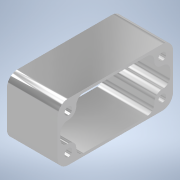
# Autodesk Inventor part: NASA-20-MM-MP-01
Saved by Autodesk Inventor 2020 (Build 240168000, 168)
## iProperties
Created: 2019-09-22
Part Number: NASA-20-MM-MP-01
Material: Aluminum 6061
Document SubType Name: Modeling
Designer: Rick Szalay
Density: 2.7 g/cm^3
Appearance: Aluminum - Flat
Description: MOUNTING BLOCK
Author: Rick Szalay
Autodesk Inventor part; units mm, degrees
ref_plane "YZ Plane" through (0, 0, 0) normal (1, 0, 0) x (0, 1, 0)
ref_plane "XZ Plane" through (0, 0, 0) normal (0, 1, 0) x (-1, 0, 0)
ref_plane "XY Plane" through (0, 0, 0) normal (0, 0, 1) x (1, 0, 0)
sketch "Sketch1" plane through (0, 0, 0) normal (1, 0, 0) x (0, 1, 0)
  line L0 (-25.4, -50.8) -> (25.4, -50.8)
  line L1 (25.4, -50.8) -> (25.4, 50.8)
  line L2 (25.4, 50.8) -> (-25.4, 50.8)
  line L3 (-25.4, 50.8) -> (-25.4, -50.8)
  line L4 (-25.4, -50.8) -> (25.4, 50.8) construction
  line L5 (25.4, -50.8) -> (-25.4, 50.8) construction
  point P0 (0, 0)
  dimension "d0" = 50.8
  dimension "d1" = 101.6
  constraints: 12 end point, 2 midpoint, 2 parallel, 1 horizontal, 1 perpendicular
  measures "d0" distance of L0.start L0.end
  measures "d1" distance between parallel lines of L2 L0
extrude "Extrusion1" add sketch "Sketch1" along normal blind 44.45
fillet "Fillet2" radius 9.525 4 edges at (22.225, 25.4, 50.8) (22.225, -25.4, 50.8) (22.225, -25.4, -50.8) (22.225, 25.4, -50.8)
sketch "Sketch5" plane through (44.45, 0, 0) normal (1, 0, 0) x (0, 0, -1)
  arc A0 (50.8, 15.875) -> (41.275, 25.4) centre (41.275, 15.875) ccw projected
  line L0 (41.275, 25.4) -> (-41.275, 25.4) projected
  arc A1 (-41.275, 25.4) -> (-50.8, 15.875) centre (-41.275, 15.875) ccw projected
  line L1 (-50.8, 15.875) -> (-50.8, -15.875) projected
  arc A2 (-50.8, -15.875) -> (-41.275, -25.4) centre (-41.275, -15.875) ccw projected
  line L2 (-41.275, -25.4) -> (41.275, -25.4) projected
  arc A3 (41.275, -25.4) -> (50.8, -15.875) centre (41.275, -15.875) ccw projected
  line L3 (50.8, -15.875) -> (50.8, 15.875) projected
  point P0 (0, 0)
hole "Hole2" at (44.45, -15.875, -41.275) at (44.45, -15.875, 41.275) at (44.45, 15.875, 41.275) at (44.45, 15.875, -41.275) direction (-1, 0, 0) diameter 6.7564 end through all clearance for "Flat Head Machine Screw (82)" size "1/4" standard "Ansi Unified Screw Threads"
sketch "Sketch6" plane through (44.45, 0, 0) normal (1, 0, 0) x (0, 0, -1)
  circle A0 centre (41.275, -15.875) radius 3.3782 projected
  circle A1 centre (41.275, -15.875) radius 6.985
  circle A2 centre (41.275, 15.875) radius 3.3782 projected
  circle A3 centre (41.275, 15.875) radius 6.985
  circle A4 centre (-41.275, 15.875) radius 3.3782 projected
  circle A5 centre (-41.275, 15.875) radius 6.985
  circle A6 centre (-41.275, -15.875) radius 3.3782 projected
  circle A7 centre (-41.275, -15.875) radius 6.985
  line L0 (-48.26, 22.86) -> (48.26, 22.86)
  line L1 (48.26, 22.86) -> (48.26, -22.86)
  line L2 (48.26, -22.86) -> (-48.26, -22.86)
  line L3 (-48.26, -22.86) -> (-48.26, 22.86)
  line L4 (-48.26, 22.86) -> (48.26, -22.86) construction
  line L5 (48.26, 22.86) -> (-48.26, -22.86) construction
  arc A8 (41.275, -25.4) -> (50.8, -15.875) centre (41.275, -15.875) ccw projected
  arc A9 (50.8, 15.875) -> (41.275, 25.4) centre (41.275, 15.875) ccw projected
  arc A10 (-41.275, 25.4) -> (-50.8, 15.875) centre (-41.275, 15.875) ccw projected
  arc A11 (-50.8, -15.875) -> (-41.275, -25.4) centre (-41.275, -15.875) ccw projected
  line L6 (50.8, -15.875) -> (50.8, 15.875) projected
  line L7 (41.275, 25.4) -> (-41.275, 25.4) projected
  point P0 (0, 0)
  point P1 (-48.26, 15.875)
  point P2 (-48.26, -15.875)
  point P3 (-41.275, -22.86)
  point P4 (41.275, -22.86)
  point P5 (48.26, -15.875)
  point P6 (48.26, 15.875)
  point P7 (41.275, 22.86)
  point P8 (-41.275, 22.86)
  dimension "d24" = 2.54
  dimension "d27" = 2.54
  constraints: 12 end point, 3 coincident, 2 horizontal, 2 midpoint, 2 parallel, 2 vertical, 1 centre point, 1 concentric, 1 perpendicular, 1 tangent, 9 other
  measures "d24" distance between parallel lines of L6 L1
  measures "d27" distance between parallel lines of L7 L0
extrude "Extrusion2" cut sketch "Sketch6" against normal through all contours A1 L2 A7 L3 A5 L0 A3 L1
fillet "Fillet3" radius 6.35 8 edges at (22.225, 15.875, 48.26) (22.225, 22.86, 41.275) (22.225, -22.86, -41.275) (22.225, -15.875, -48.26) (22.225, 15.875, -48.26) (22.225, 22.86, -41.275) (22.225, -22.86, 41.275) (22.225, -15.875, 48.26)
equation "\"d2\" = Base"
equation "\"Base\" = 44.45"
body "Solid1"
